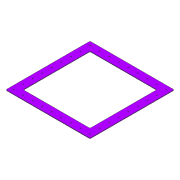
# Autodesk Inventor part: panelFrame
Saved by Autodesk Inventor 2017 (Build 210142000, 142)
## iProperties
Created: 2016-11-30
Part Number: panelFrame
Material: Generic
Document SubType Name: Modeling
Designer: krosie
Density: 1 g/cm^3
Appearance: Default
Author: krosie
Autodesk Inventor part; units mm, degrees
ref_plane "YZ Plane" through (0, 0, 0) normal (1, 0, 0) x (0, 1, 0)
ref_plane "XZ Plane" through (0, 0, 0) normal (0, 1, 0) x (-1, 0, 0)
ref_plane "XY Plane" through (0, 0, 0) normal (0, 0, 1) x (1, 0, 0)
sketch "Sketch1" plane through (0, 0, 0) normal (0, 0, 1) x (1, 0, 0)
  line L0 (-215, -220) -> (215, -220)
  line L1 (220, -215) -> (220, 215)
  line L2 (215, 220) -> (-215, 220)
  line L3 (-220, 215) -> (-220, -215)
  line L4 (-220, -220) -> (220, 220) construction
  line L5 (220, -220) -> (-220, 220) construction
  line L6 (-170, -175) -> (170, -175)
  line L7 (175, -170) -> (175, 170)
  line L8 (170, 175) -> (-170, 175)
  line L9 (-175, 170) -> (-175, -170)
  line L10 (-175, -175) -> (175, 175) construction
  line L11 (175, -175) -> (-175, 175) construction
  arc A0 (-173, 175) -> (-175, 173) centre (-173, 173) ccw
  arc A1 (-170, 175) -> (-175, 170) centre (-170, 170) ccw
  arc A2 (175, 170) -> (170, 175) centre (170, 170) ccw
  arc A3 (170, -175) -> (175, -170) centre (170, -170) ccw
  arc A4 (-175, -170) -> (-170, -175) centre (-170, -170) ccw
  arc A5 (-220, -215) -> (-215, -220) centre (-215, -215) ccw
  arc A6 (215, -220) -> (220, -215) centre (215, -215) ccw
  arc A7 (220, 215) -> (215, 220) centre (215, 215) ccw
  arc A8 (-215, 220) -> (-220, 215) centre (-215, 215) ccw
  line L12 (-200, -200) -> (-200, 200) construction
  line L13 (-200, 200) -> (200, 200) construction
  line L14 (200, 200) -> (200, -200) construction
  line L15 (200, -200) -> (-200, -200) construction
  circle A9 centre (-200, 200) radius 2.5
  circle A10 centre (-150, 200) radius 2.5
  circle A11 centre (-100, 200) radius 2.5
  circle A12 centre (-50, 200) radius 2.5
  circle A13 centre (0, 200) radius 2.5
  circle A14 centre (50, 200) radius 2.5
  circle A15 centre (100, 200) radius 2.5
  circle A16 centre (150, 200) radius 2.5
  circle A17 centre (200, 200) radius 2.5
  circle A18 centre (200, 150) radius 2.5
  circle A19 centre (200, 100) radius 2.5
  circle A20 centre (200, 50) radius 2.5
  circle A21 centre (200, 0) radius 2.5
  circle A22 centre (200, -50) radius 2.5
  circle A23 centre (200, -100) radius 2.5
  circle A24 centre (200, -150) radius 2.5
  circle A25 centre (200, -200) radius 2.5
  circle A26 centre (150, -200) radius 2.5
  circle A27 centre (100, -200) radius 2.5
  circle A28 centre (50, -200) radius 2.5
  circle A29 centre (0, -200) radius 2.5
  circle A30 centre (-50, -200) radius 2.5
  circle A31 centre (-100, -200) radius 2.5
  circle A32 centre (-150, -200) radius 2.5
  circle A33 centre (-200, -200) radius 2.5
  circle A34 centre (-200, -150) radius 2.5
  circle A35 centre (-200, -100) radius 2.5
  circle A36 centre (-200, -50) radius 2.5
  circle A37 centre (-200, 0) radius 2.5
  circle A38 centre (-200, 50) radius 2.5
  circle A39 centre (-200, 100) radius 2.5
  circle A40 centre (-200, 150) radius 2.5
  point P0 (0, 0)
  dimension "d0" = 440
  dimension "d1" = 440
  dimension "d2" = 350
  dimension "d3" = 350
  dimension "d4" = 2
  dimension "d5" = 5
  dimension "d6" = 5
  dimension "d7" = 5
  dimension "d8" = 5
  dimension "d9" = 5
  dimension "d10" = 5
  dimension "d11" = 5
  dimension "d12" = 5
  dimension "d13" = 20
  dimension "d14" = 5
  dimension "d91" = 50
  dimension "d98" = 50
  dimension "d105" = 50
  dimension "d112" = 50
  constraints: 41 centre point, 32 end point, 18 point on circle, 18 point on line, 18 tangent, 6 parallel, 4 horizontal, 4 midpoint, 3 perpendicular, 2 vertical, 1 coincident, 65 other
  measures "d0" distance of L5.end L4.end
  measures "d1" distance of L4.end L5.start
  measures "d2" distance of L11.end L10.end
  measures "d3" distance of L10.end L11.start
  measures "d4" radius of A0
  measures "d5" radius of A1
  measures "d6" radius of A2
  measures "d7" radius of A3
  measures "d8" radius of A4
  measures "d9" radius of A5
  measures "d10" radius of A6
  measures "d11" radius of A7
  measures "d12" radius of A8
  measures "d13" distance between parallel lines of L3 L12
  measures "d14" diameter of A9
  measures "d91" distance of A9.centre A10.centre
  measures "d98" distance of A17.centre A18.centre
  measures "d105" distance of A25.centre A26.centre
  measures "d112" distance of A33.centre A34.centre
extrude "Extrusion3" add sketch "Sketch1" along normal blind 3
body "Solid3"
